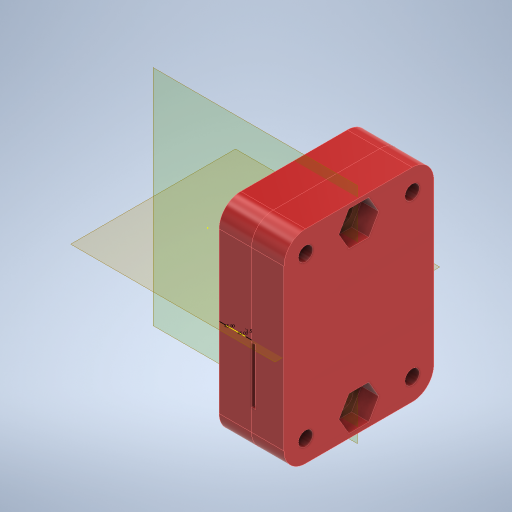
# Autodesk Inventor part: Final de Correa
Saved by Autodesk Inventor 2023 (Build 270158000, 158)
## iProperties
Created: 2023-12-12
Part Number: Final de Correa
Material: PET Plastic
Document SubType Name: Modeling
Designer: juanp
Density: 1.541 g/cm^3
Appearance: Red
Author: juanp
Autodesk Inventor part; units mm, degrees
ref_plane "XZ Plane" through (0, 0, 0) normal (0, 1, 0) x (-1, 0, 0)
ref_plane "XY Plane" through (0, 0, 0) normal (0, 0, 1) x (1, 0, 0)
sketch "Sketch1" plane through (0, 0, 0) normal (0, 1, 0) x (-1, 0, 0)
  circle A0 centre (6.85, 6.85) radius 9.6874
  circle A1 centre (6.85, 6.85) radius 2.65
  circle A2 centre (6.85, 6.85) radius 6.1
  line L0 (0.75, -48.7151) -> (0.75, 23.9132) construction
  line L1 (-0.75, -62.7525) -> (-0.75, 42.1008) construction
  circle A3 centre (-6.85, -6.85) radius 9.6874
  circle A4 centre (-6.85, -6.85) radius 2.65
  circle A5 centre (-6.85, -6.85) radius 6.1
  line L2 (-6.85, -6.85) -> (6.85, 6.85) construction
  point P0 (0, 0)
  point P1 (0, 0)
  dimension "d0" = 5.3
  dimension "d1" = 12.2
  dimension "d2" = 1.5
  dimension "d3" = 5.3
  dimension "d4" = 12.2
  dimension "d5" = 19.3747
  constraints: 6 centre point, 6 end point, 5 coincident, 3 tangent, 2 vertical, 1 equal radius, 1 midpoint
  measures "d0" diameter of A1
  measures "d1" diameter of A2
  measures "d2" distance between parallel lines of L0 L1
  measures "d3" diameter of A4
  measures "d4" diameter of A5
  measures "d5" diameter of A0
extrude "Extrusion1" add sketch "Sketch1" along normal blind 13.5 contours A2
extrude "Extrusion2" add sketch "Sketch1" against normal blind 13.5 contours A5
extrude "Extrusion3" cut sketch "Sketch1" along normal mid plane 1 contours A2 | A5
ref_plane "Work Plane1" through (20, 0, 0) normal (1, 0, 0) x (0, 1, 0)
sketch "Sketch2" plane through (20, 0, 0) normal (1, 0, 0) x (0, 1, 0)
  line L0 (0.5, 0.75) -> (0.5, 12.95) construction
  line L1 (13.5, 0.75) -> (13.5, 12.95) construction
  line L2 (-0.5, -0.75) -> (-0.5, -12.95) construction
  line L3 (-13.5, -0.75) -> (-13.5, -12.95) construction
  line L4 (0.5, 12.95) -> (13.5, 12.95) construction
  line L5 (0.5, 0.75) -> (13.5, 0.75) construction
  line L6 (-0.5, -0.75) -> (-13.5, -0.75) construction
  line L7 (-0.5, -12.95) -> (-13.5, -12.95) construction
  line L8 (13.5, 12.95) -> (0.5, 0.75) construction
  line L9 (-0.5, -0.75) -> (-13.5, -12.95) construction
  line L10 (14, 13.7) -> (0, 13.7) construction
  line L11 (0, 13.7) -> (0, 0) construction
  line L12 (0, 0) -> (14, 0) construction
  line L13 (14, 0) -> (14, 13.7) construction
  line L14 (14, 13.7) -> (0, 0) construction
  line L15 (0, 13.7) -> (14, 0) construction
  line L16 (-14, -13.7) -> (0, -13.7) construction
  line L17 (0, -13.7) -> (0, 0) construction
  line L18 (0, 0) -> (-14, 0) construction
  line L19 (-14, 0) -> (-14, -13.7) construction
  line L20 (-14, -13.7) -> (0, 0) construction
  line L21 (0, -13.7) -> (-14, 0) construction
  line L22 (7, 12.95) -> (7, 13.7) construction
  line L23 (-7, -12.95) -> (-7, -13.7) construction
  line L24 (13.5, 12.325) -> (0.5, 12.325)
  line L25 (0.5, 12.325) -> (0.5, 14.325)
  line L26 (0.5, 14.325) -> (13.5, 14.325)
  line L27 (13.5, 14.325) -> (13.5, 12.325)
  line L28 (13.5, 12.325) -> (0.5, 14.325) construction
  line L29 (0.5, 12.325) -> (13.5, 14.325) construction
  line L30 (-0.5, -12.325) -> (-13.5, -12.325)
  line L31 (-13.5, -12.325) -> (-13.5, -14.325)
  line L32 (-13.5, -14.325) -> (-0.5, -14.325)
  line L33 (-0.5, -14.325) -> (-0.5, -12.325)
  line L34 (-0.5, -12.325) -> (-13.5, -14.325) construction
  line L35 (-13.5, -12.325) -> (-0.5, -14.325) construction
  line L36 (-23.5, -17.325) -> (23.5, -17.325)
  line L37 (23.5, -17.325) -> (23.5, 17.325)
  line L38 (23.5, 17.325) -> (-23.5, 17.325)
  line L39 (-23.5, 17.325) -> (-23.5, -17.325)
  line L40 (-23.5, -17.325) -> (23.5, 17.325) construction
  line L41 (23.5, -17.325) -> (-23.5, 17.325) construction
  point P0 (7, 6.85)
  point P1 (-7, -6.85)
  point P2 (7, 13.325)
  point P3 (-7, -13.325)
  dimension "d13" = 2
  dimension "d14" = 13
  dimension "d15" = 10
  dimension "d16" = 3
  constraints: 68 end point, 18 midpoint, 13 parallel, 5 horizontal, 5 perpendicular
  measures "d13" distance between parallel lines of L24 L26
  measures "d14" distance between parallel lines of L27 L25
  measures "d15" distance between parallel lines of L37 L27
  measures "d16" distance between parallel lines of L38 L26
extrude "Extrusion4" add sketch "Sketch2" along normal blind 7.5 separate body
sketch "Sketch3" plane through (27.5, 0, 0) normal (1, 0, 0) x (0, 0, -1)
  line L0 (-12.325, 13.5) -> (-12.325, 0.5) projected
  line L1 (-12.325, 13.5) -> (17.325, 13.5)
  line L2 (17.325, 13.5) -> (17.325, 0.5)
  line L3 (17.325, 0.5) -> (-12.325, 0.5)
  line L4 (-12.325, 0.5) -> (-12.325, 13.5)
  line L5 (12.325, -13.5) -> (12.325, -0.5) projected
  line L6 (12.325, -0.5) -> (-17.325, -0.5)
  line L7 (-17.325, -0.5) -> (-17.325, -13.5)
  line L8 (-17.325, -13.5) -> (12.325, -13.5)
  line L9 (12.325, -13.5) -> (12.325, -0.5)
  line L10 (14.325, -13.5) -> (12.325, -13.5) projected
  line L11 (-12.325, 0.5) -> (-14.325, 0.5) projected
  line L12 (17.325, -23.5) -> (17.325, 23.5) projected
  point P0 (0, 0)
  point P1 (-12.325, 0.5)
  constraints: 16 end point, 5 parallel, 3 collinear, 2 horizontal, 2 perpendicular
extrude "Extrusion5" cut sketch "Sketch3" against normal blind 0.9 contours L1 L2 L3 L0 bodies 1 2
fillet "Fillet1" radius 4 2 edges at (26.6, 7, 12.325) (27.5, -7, -12.325)
fillet "Fillet2" radius 5 4 edges at (23.75, 23.5, -17.325) (23.75, 23.5, 17.325) (23.75, -23.5, 17.325) (23.75, -23.5, -17.325)
sketch "Sketch4" plane through (27.5, 0, 0) normal (1, 0, 0) x (0, 0, -1)
  line L0 (12.325, 23.5) -> (-12.325, 23.5) projected
  line L1 (17.325, -18.5) -> (17.325, 18.5) projected
  line L2 (-12.325, -23.5) -> (12.325, -23.5) projected
  line L3 (-17.325, 18.5) -> (-17.325, -18.5) projected
  line L4 (-12.325, 13.5) -> (-12.325, 0.5) projected
  line L5 (-14.325, 13.5) -> (-12.325, 13.5) projected
  line L6 (-14.325, 0.5) -> (-14.325, 13.5) projected
  line L7 (-12.325, 0.5) -> (-14.325, 0.5) projected
  line L8 (12.325, -0.5) -> (14.325, -0.5) projected
  line L9 (12.325, -13.5) -> (12.325, -0.5) projected
  line L10 (14.325, -13.5) -> (12.325, -13.5) projected
  line L11 (14.325, -0.5) -> (14.325, -13.5) projected
  arc A0 (12.325, -23.5) -> (17.325, -18.5) centre (12.325, -18.5) ccw projected
  arc A1 (-17.325, -18.5) -> (-12.325, -23.5) centre (-12.325, -18.5) ccw projected
  arc A2 (-12.325, 23.5) -> (-17.325, 18.5) centre (-12.325, 18.5) ccw projected
  arc A3 (17.325, 18.5) -> (12.325, 23.5) centre (12.325, 18.5) ccw projected
  point P0 (0, 0)
extrude "Extrusion6" add sketch "Sketch4" along normal blind 7.5 separate body contours A3 L1 A0 L2 A1 L3 A2 L0 | L4 L7 L6 L5 | L8 L11 L10 L9
sketch "Sketch5" plane through (35, 0, 0) normal (1, 0, 0) x (0, 0, -1)
  line L0 (17.325, -18.5) -> (17.325, 18.5) projected
  arc A0 (17.325, 18.5) -> (12.325, 23.5) centre (12.325, 18.5) ccw projected
  line L1 (12.325, 23.5) -> (-12.325, 23.5) projected
  arc A1 (-12.325, 23.5) -> (-17.325, 18.5) centre (-12.325, 18.5) ccw projected
  line L2 (-17.325, 18.5) -> (-17.325, -18.5) projected
  arc A2 (-17.325, -18.5) -> (-12.325, -23.5) centre (-12.325, -18.5) ccw projected
  line L3 (-12.325, -23.5) -> (12.325, -23.5) projected
  arc A3 (12.325, -23.5) -> (17.325, -18.5) centre (12.325, -18.5) ccw projected
  circle A4 centre (-12.325, 18.5) radius 1.65
  circle A5 centre (12.325, 18.5) radius 1.65
  circle A6 centre (-12.325, -18.5) radius 1.65
  circle A7 centre (12.325, -18.5) radius 1.65
  line L4 (-12.325, 18.5) -> (12.325, 18.5) construction
  line L5 (12.325, -18.5) -> (-12.325, -18.5) construction
  circle A8 centre (0, 18.5) radius 2.65
  circle A9 centre (0, -18.5) radius 2.65
  point P0 (0, 0)
  dimension "d25" = 3.3
  dimension "d28" = 5.3
  dimension "d29" = 5.3
  constraints: 6 centre point, 4 coincident, 4 end point, 3 equal radius, 2 horizontal, 2 midpoint
  measures "d25" diameter of A6
  measures "d28" diameter of A8
  measures "d29" diameter of A9
extrude "Extrusion7" cut sketch "Sketch5" against normal through all contours A4 | A5 | A6 | A7 | A8 | A9 bodies 3 2
ref_plane "Work Plane2" through (27.5, -18.5, 0) normal (0, 0, -1) x (-1, 0, 0)
ref_plane "Work Plane3" through (27.5, 0, 12.325) normal (0, 1, 0) x (1, 0, 0)
sketch "Sketch7" plane through (35, 0, 0) normal (1, 0, 0) x (0, 0, -1)
  circle A0 centre (12.325, -18.5) radius 1.65 projected
  circle A1 centre (-12.325, 18.5) radius 1.65 projected
  circle A2 centre (0, -18.5) radius 2.65 projected
  circle A3 centre (-12.325, -18.5) radius 1.65 projected
  circle A4 centre (12.325, 18.5) radius 1.65 projected
  circle A5 centre (0, 18.5) radius 2.65 projected
  line L0 (17.325, -18.5) -> (17.325, 18.5) projected
  arc A6 (17.325, 18.5) -> (12.325, 23.5) centre (12.325, 18.5) ccw projected
  line L1 (12.325, 23.5) -> (-12.325, 23.5) projected
  arc A7 (-12.325, 23.5) -> (-17.325, 18.5) centre (-12.325, 18.5) ccw projected
  line L2 (-17.325, 18.5) -> (-17.325, -18.5) projected
  arc A8 (-17.325, -18.5) -> (-12.325, -23.5) centre (-12.325, -18.5) ccw projected
  line L3 (-12.325, -23.5) -> (12.325, -23.5) projected
  arc A9 (12.325, -23.5) -> (17.325, -18.5) centre (12.325, -18.5) ccw projected
  line L4 (2.3094, 22.5) -> (4.6188, 18.5)
  line L5 (4.6188, 18.5) -> (2.3094, 14.5)
  line L6 (2.3094, 14.5) -> (-2.3094, 14.5)
  line L7 (-2.3094, 14.5) -> (-4.6188, 18.5)
  line L8 (-4.6188, 18.5) -> (-2.3094, 22.5)
  line L9 (-2.3094, 22.5) -> (2.3094, 22.5)
  line L10 (2.3094, -14.5) -> (4.6188, -18.5)
  line L11 (4.6188, -18.5) -> (2.3094, -22.5)
  line L12 (2.3094, -22.5) -> (-2.3094, -22.5)
  line L13 (-2.3094, -22.5) -> (-4.6188, -18.5)
  line L14 (-4.6188, -18.5) -> (-2.3094, -14.5)
  line L15 (-2.3094, -14.5) -> (2.3094, -14.5)
  point P0 (0, 0)
  point P1 (0, 22.5)
  dimension "d33" = 8
  constraints: 24 end point, 2 coincident, 2 horizontal, 1 midpoint, 1 parallel, 26 other
  measures "d33" distance from line of point (0, 22.5) L6
extrude "Extrusion9" cut sketch "Sketch7" against normal blind 4 contours L4 L5 L6 L7 L8 L9 | L10 L11 L12 L13 L14 L15 bodies 3
sketch "Sketch8" plane through (27.5, 0, 0) normal (1, 0, 0) x (0, 0, -1)
  line L0 (-17.3385, -0.5) -> (8.325, -0.5)
  line L1 (-8.325, 0.5) -> (-8.325, 13.5) projected
  line L2 (17.325, 0.5) -> (-8.325, 0.5) construction
  line L3 (17.325, 13.5) -> (17.325, 0.5) projected
  line L4 (-8.325, 13.5) -> (17.325, 13.5) construction
  line L5 (-8.325, 13.5) -> (-7.505, 13.5)
  line L6 (-7.505, 13.5) -> (-7.505, 0.5)
  line L7 (-7.505, 0.5) -> (-8.325, 0.5)
  line L8 (-8.325, 0.5) -> (-8.325, 13.5)
  line L9 (8.325, -0.5) -> (7.505, -0.5)
  line L10 (7.505, -0.5) -> (7.505, -13.5)
  line L11 (7.505, -13.5) -> (8.325, -13.5)
  line L12 (8.325, -13.5) -> (8.325, -0.5)
  line L13 (-6.325, 13.5) -> (-5.505, 13.5)
  line L14 (-5.505, 13.5) -> (-5.505, 0.5)
  line L15 (-5.505, 0.5) -> (-6.325, 0.5)
  line L16 (-6.325, 0.5) -> (-6.325, 13.5)
  line L17 (-4.325, 13.5) -> (-3.505, 13.5)
  line L18 (-3.505, 13.5) -> (-3.505, 0.5)
  line L19 (-3.505, 0.5) -> (-4.325, 0.5)
  line L20 (-4.325, 0.5) -> (-4.325, 13.5)
  line L21 (-2.325, 13.5) -> (-1.505, 13.5)
  line L22 (-1.505, 13.5) -> (-1.505, 0.5)
  line L23 (-1.505, 0.5) -> (-2.325, 0.5)
  line L24 (-2.325, 0.5) -> (-2.325, 13.5)
  line L25 (-0.325, 13.5) -> (0.495, 13.5)
  line L26 (0.495, 13.5) -> (0.495, 0.5)
  line L27 (0.495, 0.5) -> (-0.325, 0.5)
  line L28 (-0.325, 0.5) -> (-0.325, 13.5)
  line L29 (1.675, 13.5) -> (2.495, 13.5)
  line L30 (2.495, 13.5) -> (2.495, 0.5)
  line L31 (2.495, 0.5) -> (1.675, 0.5)
  line L32 (1.675, 0.5) -> (1.675, 13.5)
  line L33 (3.675, 13.5) -> (4.495, 13.5)
  line L34 (4.495, 13.5) -> (4.495, 0.5)
  line L35 (4.495, 0.5) -> (3.675, 0.5)
  line L36 (3.675, 0.5) -> (3.675, 13.5)
  line L37 (5.675, 13.5) -> (6.495, 13.5)
  line L38 (6.495, 13.5) -> (6.495, 0.5)
  line L39 (6.495, 0.5) -> (5.675, 0.5)
  line L40 (5.675, 0.5) -> (5.675, 13.5)
  line L41 (7.675, 13.5) -> (8.495, 13.5)
  line L42 (8.495, 13.5) -> (8.495, 0.5)
  line L43 (8.495, 0.5) -> (7.675, 0.5)
  line L44 (7.675, 0.5) -> (7.675, 13.5)
  line L45 (9.675, 13.5) -> (10.495, 13.5)
  line L46 (10.495, 13.5) -> (10.495, 0.5)
  line L47 (10.495, 0.5) -> (9.675, 0.5)
  line L48 (9.675, 0.5) -> (9.675, 13.5)
  line L49 (6.325, -0.5) -> (5.505, -0.5)
  line L50 (5.505, -0.5) -> (5.505, -13.5)
  line L51 (5.505, -13.5) -> (6.325, -13.5)
  line L52 (6.325, -13.5) -> (6.325, -0.5)
  line L53 (4.325, -0.5) -> (3.505, -0.5)
  line L54 (3.505, -0.5) -> (3.505, -13.5)
  line L55 (3.505, -13.5) -> (4.325, -13.5)
  line L56 (4.325, -13.5) -> (4.325, -0.5)
  line L57 (2.325, -0.5) -> (1.505, -0.5)
  line L58 (1.505, -0.5) -> (1.505, -13.5)
  line L59 (1.505, -13.5) -> (2.325, -13.5)
  line L60 (2.325, -13.5) -> (2.325, -0.5)
  line L61 (0.325, -0.5) -> (-0.495, -0.5)
  line L62 (-0.495, -0.5) -> (-0.495, -13.5)
  line L63 (-0.495, -13.5) -> (0.325, -13.5)
  line L64 (0.325, -13.5) -> (0.325, -0.5)
  line L65 (-1.675, -0.5) -> (-2.495, -0.5)
  line L66 (-2.495, -0.5) -> (-2.495, -13.5)
  line L67 (-2.495, -13.5) -> (-1.675, -13.5)
  line L68 (-1.675, -13.5) -> (-1.675, -0.5)
  line L69 (-3.675, -0.5) -> (-4.495, -0.5)
  line L70 (-4.495, -0.5) -> (-4.495, -13.5)
  line L71 (-4.495, -13.5) -> (-3.675, -13.5)
  line L72 (-3.675, -13.5) -> (-3.675, -0.5)
  line L73 (-5.675, -0.5) -> (-6.495, -0.5)
  line L74 (-6.495, -0.5) -> (-6.495, -13.5)
  line L75 (-6.495, -13.5) -> (-5.675, -13.5)
  line L76 (-5.675, -13.5) -> (-5.675, -0.5)
  line L77 (-7.675, -0.5) -> (-8.495, -0.5)
  line L78 (-8.495, -0.5) -> (-8.495, -13.5)
  line L79 (-8.495, -13.5) -> (-7.675, -13.5)
  line L80 (-7.675, -13.5) -> (-7.675, -0.5)
  line L81 (-9.675, -0.5) -> (-10.495, -0.5)
  line L82 (-10.495, -0.5) -> (-10.495, -13.5)
  line L83 (-10.495, -13.5) -> (-9.675, -13.5)
  line L84 (-9.675, -13.5) -> (-9.675, -0.5)
  line L85 (-11.675, -0.5) -> (-12.495, -0.5)
  line L86 (-12.495, -0.5) -> (-12.495, -13.5)
  line L87 (-12.495, -13.5) -> (-11.675, -13.5)
  line L88 (-11.675, -13.5) -> (-11.675, -0.5)
  line L89 (-13.675, -0.5) -> (-14.495, -0.5)
  line L90 (-14.495, -0.5) -> (-14.495, -13.5)
  line L91 (-14.495, -13.5) -> (-13.675, -13.5)
  line L92 (-13.675, -13.5) -> (-13.675, -0.5)
  line L93 (-15.675, -0.5) -> (-16.495, -0.5)
  line L94 (-16.495, -0.5) -> (-16.495, -13.5)
  line L95 (-16.495, -13.5) -> (-15.675, -13.5)
  line L96 (-15.675, -13.5) -> (-15.675, -0.5)
  line L97 (-17.675, -0.5) -> (-18.495, -0.5)
  line L98 (-18.495, -0.5) -> (-18.495, -13.5)
  line L99 (-18.495, -13.5) -> (-17.675, -13.5)
  line L100 (-17.675, -13.5) -> (-17.675, -0.5)
  line L101 (-19.675, -0.5) -> (-20.495, -0.5)
  line L102 (-20.495, -0.5) -> (-20.495, -13.5)
  line L103 (-20.495, -13.5) -> (-19.675, -13.5)
  line L104 (-19.675, -13.5) -> (-19.675, -0.5)
  line L105 (11.675, 13.5) -> (12.495, 13.5)
  line L106 (12.495, 13.5) -> (12.495, 0.5)
  line L107 (12.495, 0.5) -> (11.675, 0.5)
  line L108 (11.675, 0.5) -> (11.675, 13.5)
  line L109 (13.675, 13.5) -> (14.495, 13.5)
  line L110 (14.495, 13.5) -> (14.495, 0.5)
  line L111 (14.495, 0.5) -> (13.675, 0.5)
  line L112 (13.675, 0.5) -> (13.675, 13.5)
  line L113 (15.675, 13.5) -> (16.495, 13.5)
  line L114 (16.495, 13.5) -> (16.495, 0.5)
  line L115 (16.495, 0.5) -> (15.675, 0.5)
  line L116 (15.675, 0.5) -> (15.675, 13.5)
  line L117 (17.675, 13.5) -> (18.495, 13.5)
  line L118 (18.495, 13.5) -> (18.495, 0.5)
  line L119 (18.495, 0.5) -> (17.675, 0.5)
  line L120 (17.675, 0.5) -> (17.675, 13.5)
  line L121 (19.675, 13.5) -> (20.495, 13.5)
  line L122 (20.495, 13.5) -> (20.495, 0.5)
  line L123 (20.495, 0.5) -> (19.675, 0.5)
  line L124 (19.675, 0.5) -> (19.675, 13.5)
  circle A0 centre (12.325, -18.5) radius 1.65 projected
  circle A1 centre (-12.325, 18.5) radius 1.65 projected
  circle A2 centre (0, -18.5) radius 2.65 projected
  circle A3 centre (-12.325, -18.5) radius 1.65 projected
  circle A4 centre (12.325, 18.5) radius 1.65 projected
  circle A5 centre (0, 18.5) radius 2.65 projected
  line L125 (8.325, -0.5) -> (14.325, -0.5) projected
  line L126 (14.325, -0.5) -> (14.325, -13.5) projected
  line L127 (14.325, -13.5) -> (8.325, -13.5) projected
  line L128 (8.325, -0.5) -> (8.325, -13.5) projected
  arc A6 (12.325, -23.5) -> (17.325, -18.5) centre (12.325, -18.5) ccw projected
  line L129 (17.325, -18.5) -> (17.325, 0.5) projected
  line L130 (17.325, 0.5) -> (-14.325, 0.5) projected
  line L131 (-14.325, 0.5) -> (-14.325, 13.5) projected
  line L132 (-14.325, 13.5) -> (17.325, 13.5) projected
  line L133 (17.325, 13.5) -> (17.325, 18.5) projected
  arc A7 (17.325, 18.5) -> (12.325, 23.5) centre (12.325, 18.5) ccw projected
  line L134 (12.325, 23.5) -> (-12.325, 23.5) projected
  arc A8 (-12.325, 23.5) -> (-17.325, 18.5) centre (-12.325, 18.5) ccw projected
  line L135 (-17.325, 18.5) -> (-17.325, -18.5) projected
  arc A9 (-17.325, -18.5) -> (-12.325, -23.5) centre (-12.325, -18.5) ccw projected
  line L136 (-12.325, -23.5) -> (12.325, -23.5) projected
  line L137 (8.325, -13.5) -> (-17.325, -13.5)
  line L138 (-17.325, 18.5) -> (-17.325, -18.5) projected
  point P0 (0, 0)
  point P1 (11.675, 0.5)
  point P2 (13.675, 0.5)
  point P3 (15.675, 0.5)
  point P4 (17.675, 0.5)
  point P5 (19.675, 0.5)
  point P6 (-17.325, -13.5)
  point P7 (-17.325, -0.5)
  dimension "d36" = 0.82
  dimension "d39" = 2
  dimension "d44" = 1.18
  dimension "d47" = 2
  constraints: 240 end point, 56 horizontal alignment, 33 parallel, 28 collinear, 3 horizontal, 2 coincident, 2 perpendicular, 2 point on line, 1 vertical, 132 other
  measures "d36" distance between parallel lines of L1 L6
  measures "d39" distance of L1.end L13.start
  measures "d44" distance between parallel lines of L16 L6
  measures "d47" distance of L10.end L50.end
extrude "Extrusion10" add sketch "Sketch8" against normal up to surface (0.9 mm away) contours L114 L115 L116 L113 | L110 L111 L112 L109 | L106 L107 L108 L105 | L46 L47 L48 L45 | L42 L43 L44 L41 | L38 L39 L40 L37 | L34 L35 L36 L33 | L30 L31 L32 L29 | L26 L27 L28 L25 | L22 L23 L24 L21 | L18 L19 L20 L17 | L14 L15 L16 L13 | L6 L7 L1 L5 bodies 2
extrude "Extrusion11" cut sketch "Sketch8" along normal blind 0.9 contours L94 L137 L135 L0 | L0 L90 L137 L96 | L0 L86 L137 L92 | L0 L82 L137 L88 | L0 L78 L137 L84 | L0 L74 L137 L80 | L0 L70 L137 L76 | L0 L66 L137 L72 | L0 L62 L137 L68 | L0 L58 L137 L64 | L0 L54 L137 L60 | L0 L50 L137 L56 | L0 L10 L137 L52 bodies 2 3
sketch "Sketch9" plane through (27.5, 0, 12.325) normal (0, 1, 0) x (1, 0, 0)
  line L0 (0, -5) -> (-7.5, -5) projected
  line L1 (0, 0) -> (0, -5) projected
  line L2 (0, -5) -> (-1.5, -5)
  line L3 (-1.5, -5) -> (-3, -3.5)
  line L4 (-3, -3.5) -> (-4.5, -3.5)
  line L5 (-4.5, -3.5) -> (-6, -5)
  line L6 (-6, -5) -> (-7.5, -5)
  point P0 (-27.5, 12.325)
  dimension "d56" = 45
  dimension "d57" = 45
  dimension "d58" = 1.5
  constraints: 10 end point, 3 parallel, 2 point on line, 1 collinear
  measures "d56" angle of L0 L3
  measures "d57" angle of L0 L5
  measures "d58" distance between parallel lines of L4 L0
body "Solid1"
body "Solid2"
body "Solid3"
